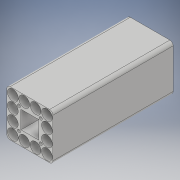
# Autodesk Inventor part: WeightHolder
Saved by Autodesk Inventor 2019.3 (Build 233278000, 278)
## iProperties
Created: 2019-07-14
Part Number: WeightHolder
Material: Generic
Document SubType Name: Modeling
Designer: mark
Density: 1 g/cm^3
Appearance: Default
Author: mark
Autodesk Inventor part; units mm, degrees
ref_plane "YZ Plane" through (0, 0, 0) normal (1, 0, 0) x (0, 1, 0)
ref_plane "XZ Plane" through (0, 0, 0) normal (0, 1, 0) x (-1, 0, 0)
ref_plane "XY Plane" through (0, 0, 0) normal (0, 0, 1) x (1, 0, 0)
sketch "Sketch1" plane through (0, 0, 0) normal (0, 0, 1) x (1, 0, 0)
  line L0 (0, 26.67) -> (26.67, 26.67)
  line L1 (26.67, 26.67) -> (26.67, 0)
  line L2 (26.67, 0) -> (0, 0)
  line L3 (0, 0) -> (0, 26.67)
  line L4 (47.835, -21.165) -> (47.835, 47.835)
  line L5 (47.835, 47.835) -> (-21.165, 47.835)
  line L6 (-21.165, 47.835) -> (-21.165, -21.165)
  line L7 (-21.165, -21.165) -> (47.835, -21.165)
  dimension "d0" = 26.67
  dimension "d16" = 69
  constraints: 16 end point, 2 horizontal, 1 coincident, 1 perpendicular, 1 vertical, 3 other
  measures "d0" distance between parallel lines of L1 L3
  measures "d16" distance between parallel lines of L4 L6
extrude "Extrusion1" add sketch "Sketch1" along normal blind 2
sketch "Sketch2" plane through (0, 0, 2) normal (0, 0, 1) x (1, 0, 0)
  circle A0 centre (4.835, 38.835) radius 8.0375
  circle A1 centre (-12.165, 38.835) radius 8.0375
  circle A2 centre (21.835, 38.835) radius 8.0375
  circle A3 centre (38.835, 38.835) radius 8.0375
  line L0 (47.835, 47.835) -> (-21.165, 47.835) projected
  line L1 (-21.165, 47.835) -> (-21.165, -21.165) projected
  circle A4 centre (-12.165, 21.835) radius 8.0375
  circle A5 centre (-12.165, 4.835) radius 8.0375
  circle A6 centre (38.835, 21.835) radius 8.0375
  circle A7 centre (38.835, 4.835) radius 8.0375
  circle A8 centre (4.835, -12.165) radius 8.0375
  circle A9 centre (-12.165, -12.165) radius 8.0375
  circle A10 centre (21.835, -12.165) radius 8.0375
  circle A11 centre (38.835, -12.165) radius 8.0375
  line L2 (47.835, -21.165) -> (47.835, 47.835) projected
  line L3 (-21.165, -21.165) -> (47.835, -21.165) projected
  line L4 (0, 0) -> (0, 26.67) projected
  line L5 (0, 26.67) -> (26.67, 26.67) projected
  line L6 (26.67, 26.67) -> (26.67, 0) projected
  line L7 (26.67, 0) -> (0, 0) projected
  point P0 (48.835, 48.835)
  point P1 (-20.165, 48.835)
  dimension "d4" = 16.075
  dimension "d5" = 16.075
  dimension "d6" = 16.075
  dimension "d7" = 16.075
  dimension "d8" = 9
  dimension "d9" = 9
  dimension "d10" = 9
  dimension "d11" = 9
  dimension "d12" = 9
  dimension "d13" = 17
  dimension "d14" = 17
  dimension "d15" = 17
  dimension "d17" = 16.075
  dimension "d18" = 16.075
  dimension "d19" = 16.075
  dimension "d20" = 16.075
  dimension "d21" = 16.075
  dimension "d22" = 16.075
  dimension "d23" = 16.075
  dimension "d24" = 16.075
  dimension "d25" = 17
  dimension "d26" = 17
  dimension "d27" = 17
  dimension "d28" = 17
  dimension "d29" = 17
  dimension "d30" = 17
  dimension "d31" = 17
  dimension "d32" = 17
  dimension "d33" = 17
  dimension "d34" = 9
  dimension "d35" = 9
  dimension "d36" = 9
  dimension "d37" = 9
  dimension "d38" = 9
  dimension "d39" = 9
  dimension "d40" = 9
  constraints: 12 centre point
  measures "d4" diameter of A0
  measures "d5" diameter of A1
  measures "d6" diameter of A2
  measures "d7" diameter of A3
  measures "d8" distance from line of L0 A1.centre
  measures "d9" distance from line of L1 A1.centre
  measures "d10" distance from line of L0 A0.centre
  measures "d11" distance from line of A2.centre L0
  measures "d12" distance from line of A3.centre L0
  measures "d13" distance of A0.centre A1.centre
  measures "d14" distance of A0.centre A2.centre
  measures "d15" distance of A2.centre A3.centre
  measures "d17" diameter of A4
  measures "d18" diameter of A5
  measures "d19" diameter of A6
  measures "d20" diameter of A7
  measures "d21" diameter of A8
  measures "d22" diameter of A9
  measures "d23" diameter of A10
  measures "d24" diameter of A11
  measures "d25" distance of A8.centre A9.centre
  measures "d26" distance of A8.centre A10.centre
  measures "d27" distance of A10.centre A11.centre
  measures "d28" distance of A4.centre A1.centre
  measures "d29" distance of A5.centre A4.centre
  measures "d30" distance of A9.centre A5.centre
  measures "d31" distance of A6.centre A3.centre
  measures "d32" distance of A6.centre A7.centre
  measures "d33" distance of A11.centre A7.centre
  measures "d34" distance from line of L2 A6.centre
  measures "d35" distance from line of L2 A7.centre
  measures "d36" distance from line of L2 A11.centre
  measures "d37" distance from line of L3 A10.centre
  measures "d38" distance from line of A8.centre L3
  measures "d39" distance from line of L3 A9.centre
  measures "d40" distance from line of L1 A5.centre
extrude "Extrusion2" add sketch "Sketch2" along normal blind 177.8
sketch "Sketch3" plane through (0, 0, 179.8) normal (0, 0, 1) x (1, 0, 0)
  circle A0 centre (-3, 29.67) radius 2.25
  circle A1 centre (29.67, 29.67) radius 2.25
  circle A2 centre (29.67, -3) radius 2.25
  circle A3 centre (-3, -3) radius 2.25
  line L0 (0, 0) -> (0, 26.67) projected
  line L1 (0, 26.67) -> (26.67, 26.67) projected
  line L2 (26.67, 26.67) -> (26.67, 0) projected
  line L3 (26.67, 0) -> (0, 0) projected
  dimension "d43" = 4.5
  dimension "d44" = 3
  dimension "d45" = 3
  dimension "d46" = 3
  dimension "d47" = 3
  dimension "d48" = 3
  dimension "d49" = 3
  dimension "d50" = 3
  dimension "d51" = 3
  constraints: 4 centre point, 3 equal radius
  measures "d43" diameter of A0
  measures "d44" distance from line of L0 A0.centre
  measures "d45" distance from line of L1 A0.centre
  measures "d46" distance from line of L1 A1.centre
  measures "d47" distance from line of L2 A1.centre
  measures "d48" distance from line of L2 A2.centre
  measures "d49" distance from line of L3 A2.centre
  measures "d50" distance from line of L3 A3.centre
  measures "d51" distance from line of A3.centre L0
extrude "Extrusion3" cut sketch "Sketch3" against normal blind 15 contours A0 | A1 | A2 | A3
fillet "Fillet1" radius 5 4 edges at (-21.165, -21.165, 89.9) (-21.165, 47.835, 89.9) (47.835, 47.835, 89.9) (47.835, -21.165, 89.9)
body "Solid1"
